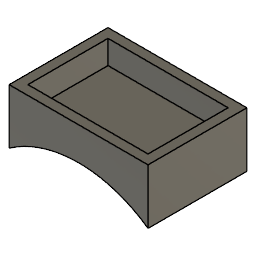
MCP3008_Halter (Autodesk Fusion 360 design; units mm, degrees)
Autodesk Fusion 360 part; units mm, degrees
box "Grundkörper Quader1" add length 17 width 25.5 height 5 placed x (0, -1, 0) y (1, 0, 0) z (0, 0, 1) at (0, 0, 0) makes body 1
shell "Schale1" thickness 2 outward yes removed faces 1 at (17, -5.6667, 5) on bodies 1
extrude "Extrusion2" add 1 faces at (17.6667, -5, -2) along direction (0, 0, -1) blind 5 on bodies 1 bodies 1
sketch "Skizze2" plane through (0, -19, 0) normal (0, -1, 0) x (1, 0, 0)
  line L0 (-2, 5) -> (-2, -7)
  line L1 (27.5, -7) -> (27.5, 5)
  line L2 (27.5, 5) -> (-2, 5)
  circle A0 centre (12.75, -27.5) radius 20.5
  line L3 (-2, -7) -> (27.5, -7)
  dimension "d9" = 41
  dimension "d16" = 20.5
  measures "d9" diameter of A0
  measures "d16" distance of A0.centre L3
extrude "Extrusion1" add sketch "Skizze2" against normal blind 21 separate body contours A0 makes body 2
shell "Schale2" thickness 5 outward yes removed faces 2 at (16.7092, -19, -31.7488) at (16.7092, 2, -31.7488) on bodies 2
combine "Kombinieren1" operation cut target body 1 tool bodies 2
equation "d16 = d9 / 2"
